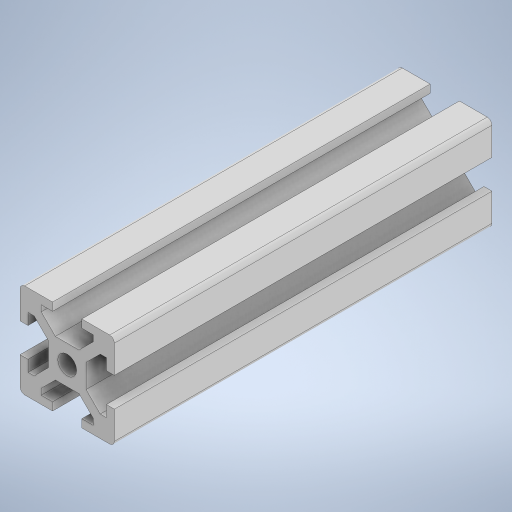
# Autodesk Inventor part: Aluminum_Profile_202090
Saved by Autodesk Inventor 2023 (Build 270158000, 158)
## iProperties
Created: 2024-02-04
Part Number: Aluminum_Profile_202090
Material: Generic
Document SubType Name: Modeling
Designer: victo
Density: 1 g/cm^3
Appearance: Default
Author: victo
Autodesk Inventor part; units mm, degrees
ref_plane "YZ Plane" through (0, 0, 0) normal (1, 0, 0) x (0, 1, 0)
ref_plane "XZ Plane" through (0, 0, 0) normal (0, 1, 0) x (-1, 0, 0)
ref_plane "XY Plane" through (0, 0, 0) normal (0, 0, 1) x (1, 0, 0)
sketch "Sketch1" plane through (0, 0, 0) normal (0, 0, 1) x (1, 0, 0)
  line L0 (-9, 10) -> (9, 10)
  line L1 (10, 9) -> (10, -9)
  line L2 (9, -10) -> (-9, -10)
  line L3 (-10, -9) -> (-10, 9)
  line L4 (-10, 10) -> (10, -10) construction
  line L5 (10, 10) -> (-10, -10) construction
  circle A0 centre (0, 0) radius 2
  line L6 (-4, 4) -> (4, 4)
  line L7 (4, 4) -> (4, -4)
  line L8 (4, -4) -> (-4, -4)
  line L9 (-4, -4) -> (-4, 4)
  line L10 (-4, 4) -> (4, -4) construction
  line L11 (4, 4) -> (-4, -4) construction
  arc A1 (-9, 10) -> (-10, 9) centre (-9, 9) ccw
  arc A2 (10, 9) -> (9, 10) centre (9, 9) ccw
  arc A3 (9, -10) -> (10, -9) centre (9, -9) ccw
  arc A4 (-10, -9) -> (-9, -10) centre (-9, -9) ccw
  line L12 (-3.1, 10) -> (3.1, 10)
  line L13 (3.1, 10) -> (3.1, -10)
  line L14 (3.1, -10) -> (-3.1, -10)
  line L15 (-3.1, -10) -> (-3.1, 10)
  line L16 (-10, 3.1) -> (10, 3.1)
  line L17 (10, 3.1) -> (10, -3.1)
  line L18 (10, -3.1) -> (-10, -3.1)
  line L19 (-10, -3.1) -> (-10, 3.1)
  line L20 (-5.5, 10) -> (5.5, 10)
  line L21 (5.5, 10) -> (5.5, -10)
  line L22 (5.5, -10) -> (-5.5, -10)
  line L23 (-5.5, -10) -> (-5.5, 10)
  line L24 (-10, 5.5) -> (10, 5.5)
  line L25 (10, 5.5) -> (10, -5.5)
  line L26 (10, -5.5) -> (-10, -5.5)
  line L27 (-10, -5.5) -> (-10, 5.5)
  line L28 (-8.3, 5.5) -> (-8.3, 3.1)
  line L29 (-8.3, -5.5) -> (-8.3, -3.1)
  line L30 (8.3, -5.5) -> (8.3, -3.1)
  line L31 (8.3, 5.5) -> (8.3, 3.1)
  line L32 (-5.5, 8.3) -> (-3.1, 8.3)
  line L33 (3.1, 8.3) -> (5.5, 8.3)
  line L34 (-5.5, -8.3) -> (-3.1, -8.3)
  line L35 (3.1, -8.3) -> (5.5, -8.3)
  line L36 (-4, 2.5) -> (-7, 5.5)
  line L37 (-4, 2.5) -> (0.2426, 2.5) construction
  line L38 (-4, -2.5) -> (-7, -5.5)
  line L39 (-4, -2.5) -> (0.2426, -2.5) construction
  line L40 (-2.5, 4) -> (-5.5, 7)
  line L41 (-2.5, 4) -> (1.7426, 4) construction
  line L42 (5.5, 7) -> (2.5, 4)
  line L43 (5.5, 7) -> (9.7426, 7) construction
  line L44 (7, 5.5) -> (4, 2.5)
  line L45 (7, 5.5) -> (11.2426, 5.5) construction
  line L46 (7, -5.5) -> (4, -2.5)
  line L47 (7, -5.5) -> (11.2426, -5.5) construction
  line L48 (2.5, -4) -> (5.5, -7)
  line L49 (2.5, -4) -> (6.7426, -4) construction
  line L50 (-2.5, -4) -> (-5.5, -7)
  line L51 (-2.5, -4) -> (1.7426, -4) construction
  point P0 (3.1, -3.1)
  point P1 (3.1, -5.5)
  point P2 (5.5, -5.5)
  point P3 (10, 3.1)
  point P4 (-5.5, -5.5)
  point P5 (-3.1, -5.5)
  point P6 (-3.1, -3.1)
  dimension "d0" = 20
  dimension "d1" = 20
  dimension "d2" = 4
  dimension "d3" = 8
  dimension "d4" = 8
  dimension "d5" = 1
  dimension "d6" = 6.2
  dimension "d7" = 3.1
  dimension "d8" = 6.2
  dimension "d9" = 3.1
  dimension "d10" = 11
  dimension "d11" = 5.5
  dimension "d12" = 11
  dimension "d13" = 5.5
  dimension "d14" = 4.3
  dimension "d15" = 4.3
  dimension "d16" = 4.3
  dimension "d17" = 4.3
  dimension "d18" = 135
  dimension "d19" = 135
  dimension "d20" = 135
  dimension "d21" = 135
  dimension "d22" = 135
  dimension "d23" = 135
  dimension "d24" = 1.3
  dimension "d25" = 1.3
  dimension "d26" = 1.3
  dimension "d27" = 1.3
  dimension "d28" = 1.3
  dimension "d29" = 1.3
  dimension "d32" = 45
  dimension "d33" = 135
  dimension "d34" = 1.3
  dimension "d35" = 1.3
  constraints: 104 end point, 56 point on line, 14 horizontal, 12 parallel, 10 perpendicular, 8 equal length, 8 point on circle, 8 tangent, 5 centre point, 4 midpoint, 3 equal radius, 1 coincident
  measures "d0" distance of L4.end L5.end
  measures "d1" distance of L5.start L4.end
  measures "d2" diameter of A0
  measures "d3" distance of L7.end L8.end
  measures "d4" distance of L6.end L7.end
  measures "d5" radius of A1
  measures "d6" distance between parallel lines of L18 L16
  measures "d7" distance from line of A0.centre L18
  measures "d8" distance between parallel lines of L15 L13
  measures "d9" distance from line of point (0, 0) L13
  measures "d10" distance between parallel lines of L23 L21
  measures "d11" distance from line of A0.centre L21
  measures "d12" distance between parallel lines of L26 L24
  measures "d13" distance from line of point (0, 0) L26
  measures "d14" distance between parallel lines of L28 L9
  measures "d15" distance between parallel lines of L7 L31
  measures "d16" distance between parallel lines of L32 L6
  measures "d17" distance between parallel lines of L8 L34
  measures "d18" angle of L37 L36
  measures "d19" angle of L38 L39
  measures "d20" angle of L41 L40
  measures "d21" angle of L42 L43
  measures "d22" angle of L44 L45
  measures "d23" angle of L47 L46
  measures "d24" distance from line of L31 L44.start
  measures "d25" distance of L30.start L46.start
  measures "d26" distance of L29.start L38.end
  measures "d27" distance of L28.start L36.end
  measures "d28" distance of L32.start L40.end
  measures "d29" distance of L33.end L42.start
  measures "d32" angle of L48 L49
  measures "d33" angle of L50 L51
  measures "d34" distance of L48.end L35.end
  measures "d35" distance of L34.start L50.end
extrude "Extrusion1" add sketch "Sketch1" along normal blind 80 contours L0 L23 L24 L3 A1 | L0 L15 L32 L23 | L24 L28 L16 L3 | L0 L21 L33 L13 | L40 L24 L23 | L0 A2 L1 L24 L21 | L24 L40 L15 L6 L9 L16 L36 L23 | L23 L36 L24 | L18 L29 L26 L3 | L40 L6 L15 | L26 L23 L2 A4 L3 | L21 L24 L42 | L42 L24 L21 L44 L16 L7 L6 L13 | L13 L6 L42 | L15 L16 L9 L6 | L6 L13 L16 L15 | L16 L9 L36 | L1 L16 L31 L24 | L24 L44 L21 | L6 L7 L16 L13 | L16 L13 L18 L15 | L15 L18 L9 L16 | L38 L23 L26 | L38 L9 L18 | L18 L9 L8 L15 L50 L26 L23 L38 | L16 L7 L18 L13 | L18 L13 L8 L15 | L15 L8 L9 L18 | L23 L34 L15 L2 | L26 L50 L23 | L1 L26 L30 L18 | L44 L7 L16 | L18 L7 L8 L13 | L8 L50 L15 | L1 A3 L2 L21 L26 | L13 L48 L8 | L8 L7 L18 L46 L21 L26 L48 L13 | L7 L46 L18 | L13 L35 L21 L2 | L46 L26 L21 | L21 L48 L26
equation "\"d7\" = 0.5 * d6"
equation "\"d8\" = d6"
equation "\"d9\" = 0.5 * d6"
equation "\"d11\" = 0.5 * d10"
equation "\"d12\" = d10"
equation "\"d13\" = 0.5 * d12"
body "Solid1"
